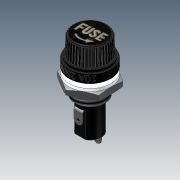
# Autodesk Inventor part: Fuse holder
Saved by Autodesk Inventor 2012 SP2 (Build 160219200, 219)
## iProperties
Created: 2017-11-11
Part Number: Fuse holder
Material: Default
Document SubType Name: Modeling
Designer: Шумейко Д.А.
Density: 1 g/cm^3
Author: Шумейко Д.А.
Autodesk Inventor part; units mm, degrees
sketch "Эскиз1" plane through (0, 0, 0) normal (0, 0, 1) x (1, 0, 0)
  circle A0 centre (0, 0) radius 5.75
  dimension "d0" = 11.5
  constraints: 1 centre point, 1 coincident
  measures "d0" diameter of A0
extrude "Выдавливание1" add sketch "Эскиз1" along normal blind 0.5
ref_plane "РабПлоскость1" through (0, 0, -6) normal (0, 0, -1) x (-1, 0, 0)
sketch "Эскиз2" plane through (0, 0, -6) normal (0, 0, -1) x (-1, 0, 0)
  circle A0 centre (0, 0) radius 6
  dimension "d4" = 12
  constraints: 1 centre point, 1 coincident
  measures "d4" diameter of A0
loft "По сечениям1" add profiles "Эскиз2" section 1 edges at (-5.75, 0, 0)
sketch "Эскиз4" plane through (0, 0, -6) normal (0, 0, -1) x (-1, 0, 0)
  circle A0 centre (0, 0) radius 7
  dimension "d9" = 14
  constraints: 1 centre point, 1 coincident
  measures "d9" diameter of A0
extrude "Выдавливание2" add sketch "Эскиз4" along normal blind 1
sketch "Эскиз5" plane through (0, 0, 0) normal (0, 0, 1) x (1, 0, 0)
  line L0 (-0.3727, 5.7711) -> (-0.0631, 6.1689)
  line L1 (0.0631, 6.1689) -> (0.3727, 5.7711)
  circle A0 centre (0, 0) radius 5.75 projected
  arc A1 (0.0631, 6.1689) -> (-0.0631, 6.1689) centre (0, 6.1198) ccw
  arc A2 (-0.4439, 5.7328) -> (0.4439, 5.7328) centre (0, 0) ccw
  arc A3 (-0.4439, 5.7328) -> (-0.3727, 5.7711) centre (-0.4516, 5.8325) ccw
  arc A4 (0.3727, 5.7711) -> (0.4439, 5.7328) centre (0.4516, 5.8325) ccw
  arc A5 (0.4439, 5.7328) -> (-0.4439, 5.7328) centre (0, 0) ccw
  point P0 (-0.4, 5.7361)
  point P1 (0, 6.25)
  point P2 (0.4, 5.7361)
  point P3 (0, 5.75)
  dimension "d12" = 0.5
  dimension "d13" = 0.8
  dimension "d14" = 0.08
  dimension "d15" = 0.1
  constraints: 16 point on circle, 6 tangent, 5 centre point, 4 end point, 4 point on line, 2 vertical alignment, 1 coincident, 1 equal length, 1 equal radius
  measures "d12" distance of point (0, 6.25) A0.start
  measures "d13" distance of point (0.4, 5.736) A0.end
  measures "d14" radius of A1
  measures "d15" radius of A3
sketch "Эскиз6" plane through (0, 0, 0) normal (1, 0, 0) x (0, 1, 0)
  line L0 (6, -6) -> (5.75, 0) projected
  point P0 (0, 0)
sweep "Сдвиг1" add profiles "Эскиз5" path "Эскиз6" contours L0 A1 L1 A4 A0 A3
sketch "Эскиз7" plane through (0, 0, -7) normal (0, 0, -1) x (-1, 0, 0)
  circle A0 centre (0, 0) radius 7 projected
  circle A1 centre (0, 0) radius 7.5
  dimension "d20" = 15
  constraints: 1 centre point, 1 coincident
  measures "d20" diameter of A1
extrude "Выдавливание3" add sketch "Эскиз7" along normal blind 3 contours A0 | A1
sketch "Эскиз8" plane through (0, 0, 0.5) normal (0, 0, 1) x (1, 0, 0)
  line L0 (-6.3909, 6.5709) -> (6.3606, 6.5709) construction
  line L1 (6.3606, 6.5709) -> (6.3606, -7.9897) construction
  line L2 (6.3606, -7.9897) -> (-6.3909, -7.9897) construction
  line L3 (-6.3909, -7.9897) -> (-6.3909, 6.5709) construction
  constraints: 1 vertical, 2 other
decal "Маркировка1"
fillet "Сопряжение1" radius 0.2 1 edges at (-5.75, 0, 0.5)
pattern_circular "Круговой массив2" count 40 over 360 about axis through (0, 0, -6) along (0, 0, 1) of "Сдвиг1"
sketch "Эскиз9" plane through (0, 0, -10) normal (0, 0, -1) x (-1, 0, 0)
  circle A0 centre (0, 0) radius 7.5 projected
  circle A1 centre (0, 0) radius 5.5
  dimension "d62" = 11
  constraints: 1 centre point, 1 coincident
  measures "d62" diameter of A1
extrude "Выдавливание4" add sketch "Эскиз9" along normal blind 9 contours A1
sketch "Эскиз10" plane through (0, 0, -19) normal (0, 0, -1) x (-1, 0, 0)
  circle A0 centre (0, 0) radius 5.5 projected
  circle A1 centre (0, 0) radius 4
  dimension "d65" = 8
  constraints: 1 centre point, 1 coincident
  measures "d65" diameter of A1
extrude "Выдавливание5" add sketch "Эскиз10" along normal blind 11 contours A1
chamfer "Фаска1" distance 0.5 angle 45 1 edges at (5.5, 0, -19)
thread "Резьба1" size "M11x1.5" class "6g" standard "ANSI Metric M Profile" full length
sketch "Эскиз11" plane through (0, 0, -30) normal (0, 0, -1) x (-1, 0, 0)
  circle A0 centre (0, 0) radius 4 projected
  line L0 (-1.9365, -3.5) -> (1.9365, -3.5)
  dimension "d73" = 3.5
  constraints: 2 end point, 2 point on circle, 1 horizontal
  measures "d73" distance from line of L0 A0.centre
extrude "Выдавливание6" cut sketch "Эскиз11" against normal blind 9 contours L0 A0 picked at (0.3981, -3.6058)
sketch "Эскиз12" plane through (0, 0, -30) normal (0, 0, -1) x (-1, 0, 0)
  arc A0 (1.9365, -3.5) -> (-1.9365, -3.5) centre (0, 0) ccw projected
  line L0 (-1.5, 2.7) -> (1.5, 2.7)
  line L1 (1.5, 2.7) -> (1.5, 2.5)
  line L2 (1.5, 2.5) -> (-1.5, 2.5)
  line L3 (-1.5, 2.5) -> (-1.5, 2.7)
  point P0 (0, 2.5)
  dimension "d76" = 0.2
  dimension "d77" = 3
  dimension "d78" = 2.5
  constraints: 8 end point, 2 parallel, 1 horizontal, 1 midpoint, 1 perpendicular, 1 vertical alignment
  measures "d76" distance of L0.end L1.end
  measures "d77" distance of L0.start L0.end
  measures "d78" distance from line of A0.centre L2
extrude "Выдавливание7" add sketch "Эскиз12" along normal blind 5
fillet "Сопряжение2" radius 1.5 2 edges at (1.5, 2.6, -35) (-1.5, 2.6, -35)
hole "Отверстие1" at (0, 2.5, -33.5) direction (0, 1, 0) diameter 1 end through all
sketch "Эскиз13" plane through (-1.9365, -3.5, -30) normal (0, -1, 0) x (1, 0, 0)
  line L0 (0, 9) -> (3.873, 9) projected
  line L1 (0.4365, 8.9) -> (3.4365, 8.9)
  line L2 (3.4365, 8.9) -> (3.4365, 8.7)
  line L3 (3.4365, 8.7) -> (0.4365, 8.7)
  line L4 (0.4365, 8.7) -> (0.4365, 8.9)
  line L5 (3.873, 9) -> (0, 9) projected
  point P0 (1.9365, 30)
  point P1 (1.9365, 8.9)
  point P2 (1.9365, 9)
  dimension "d91" = 0.2
  dimension "d92" = 3
  dimension "d93" = 0.1
  constraints: 8 end point, 2 midpoint, 2 parallel, 1 horizontal, 1 perpendicular, 1 vertical alignment
  measures "d91" distance of L1.end L2.end
  measures "d92" distance of L2.end L3.end
  measures "d93" distance between parallel lines of L0 L1
sketch "Эскиз14" plane through (0, 0, 0) normal (1, 0, 0) x (0, 1, 0)
  arc A0 (-3.5, -21.1) -> (-4.3, -21.9) centre (-3.5, -21.9) ccw
  line L0 (-4.3, -21.9) -> (-4.3, -25.9)
  point P0 (0, 0)
  dimension "d94" = 0.8
  dimension "d95" = 4
  constraints: 2 end point, 2 point on circle, 1 centre point, 1 horizontal alignment, 1 tangent, 1 vertical, 1 vertical alignment
  measures "d94" radius of A0
  measures "d95" distance of L0.start L0.end
sweep "Сдвиг2" add profiles "Эскиз13" path "Эскиз14"
fillet "Сопряжение3" radius 1.5 2 edges at (1.5, -4.2, -25.9) (-1.5, -4.2, -25.9)
hole "Отверстие2" at (0, -4.3, -24.4) direction (0, 1, 0) diameter 1 depth 0.2 tip angle 118
ref_plane "РабПлоскость2" through (0, 0, -11.5) normal (0, 0, -1) x (-1, 0, 0)
sketch "Эскиз15" plane through (0, 0, -11.5) normal (0, 0, -1) x (-1, 0, 0)
  circle A0 centre (0, 0) radius 7.5 projected
  circle A1 centre (0, 0) radius 5.5 projected
extrude "Выдавливание8" add sketch "Эскиз15" along normal blind 1
sketch "Эскиз16" plane through (0, 0, -12.5) normal (0, 0, -1) x (-1, 0, 0)
  circle A0 centre (0, 0) radius 5.5 projected
  circle A1 centre (0, 0) radius 7.5 projected
  line L0 (0, 8.6603) -> (7.5, 4.3301)
  line L1 (7.5, 4.3301) -> (7.5, -4.3301)
  line L2 (7.5, -4.3301) -> (0, -8.6603)
  line L3 (0, -8.6603) -> (-7.5, -4.3301)
  line L4 (-7.5, -4.3301) -> (-7.5, 4.3301)
  line L5 (-7.5, 4.3301) -> (0, 8.6603)
  dimension "d110" = 15
  constraints: 12 end point, 1 coincident, 1 vertical alignment, 13 other
  measures "d110" distance between parallel lines of L1 L4
extrude "Выдавливание9" add sketch "Эскиз16" along normal blind 2.5
sketch "Эскиз17" plane through (0, 0, 0) normal (1, 0, 0) x (0, 1, 0)
  line L0 (0, 0) -> (0, -44.8004)
  line L1 (8.6603, -12.5) -> (5.6603, -12.5)
  line L2 (8.6603, -15) -> (4.3301, -15) projected
  line L3 (8.6603, -12.5) -> (8.6603, -13)
  line L4 (8.6603, -13) -> (7.1603, -12.5)
  line L5 (8.6603, -12.5) -> (7.1603, -12.5)
  line L6 (8.6603, -15) -> (8.6603, -14.5)
  line L7 (8.6603, -14.5) -> (7.1603, -15)
  line L8 (8.6603, -15) -> (7.1603, -15)
  dimension "d113" = 44.8004
  dimension "d114" = 0.5
  dimension "d115" = 1.5
  dimension "d117" = 0.5
  dimension "d118" = 1.5
  constraints: 16 end point, 3 perpendicular, 1 coincident, 1 collinear, 1 horizontal, 1 midpoint, 1 point on line, 1 vertical
  measures "d113" distance of L0.end L0.start
  measures "d114" distance of L1.start L3.end
  measures "d115" distance from line of L4.end L3
  measures "d117" distance of L2.start L6.end
  measures "d118" distance from line of L7.end L6
revolve "Вращение1" cut sketch "Эскиз17" angle 360 about axis through (0, 0, 0) along (0, 0, -1)
ref_plane "РабПлоскость3" through (0, 9.25, 0) normal (0, 1, 0) x (-1, 0, 0)
sketch "Эскиз18" plane through (0, 9.25, 0) normal (0, 1, 0) x (-1, 0, 0)
  line L0 (7.588, -9.5) -> (-7.412, -9.5) construction
  line L1 (-7.412, -9.5) -> (-7.412, -7.5) construction
  line L2 (-7.412, -7.5) -> (7.588, -7.5) construction
  line L3 (7.588, -7.5) -> (7.588, -9.5) construction
  line L4 (7.5, -10) -> (-7.5, -10) projected
  line L5 (6.3092, -7.4579) -> (7.2849, -7.4579)
  line L6 (7.2849, -7.4579) -> (7.2849, -7.6621)
  line L7 (7.2849, -7.6621) -> (6.9219, -7.6621)
  line L8 (6.9219, -7.6621) -> (6.9219, -9.0024)
  line L9 (6.9219, -9.0024) -> (7.2849, -9.0024)
  line L10 (7.2849, -9.0024) -> (7.2849, -9.1856)
  spline S0 degree 2 poles (7.2849, -9.1856) (7.0791, -9.1856) (6.8846, -9.3023) (6.8716, -9.4643) knots 0 0 0 1 2 2 2
  line L11 (6.8716, -9.4643) -> (6.6642, -9.4643)
  line L12 (6.6642, -9.4643) -> (6.6642, -7.6621)
  line L13 (6.6642, -7.6621) -> (6.3092, -7.6621)
  line L14 (6.3092, -7.6621) -> (6.3092, -7.4579)
  spline S1 degree 2 poles (4.729, -8.0932) (4.729, -7.9489) (4.8214, -7.7026) (4.9057, -7.6118) knots 0 0 0 1 2 2 2
  spline S2 degree 2 poles (4.9057, -7.6118) (4.99, -7.5211) (5.2412, -7.4157) (5.3968, -7.4157) knots 0 0 0 1 2 2 2
  spline S3 degree 2 poles (5.3968, -7.4157) (5.5394, -7.4157) (5.8182, -7.4789) (5.9203, -7.5292) knots 0 0 0 1 2 2 2
  line L15 (5.9203, -7.5292) -> (5.9203, -7.8128)
  line L16 (5.9203, -7.8128) -> (5.9008, -7.8128)
  spline S4 degree 2 poles (5.9008, -7.8128) (5.87, -7.7901) (5.7549, -7.7318) (5.6853, -7.7058) knots 0 0 0 1 2 2 2
  spline S5 degree 2 poles (5.6853, -7.7058) (5.6058, -7.6783) (5.4746, -7.6475) (5.3919, -7.6475) knots 0 0 0 1 2 2 2
  spline S6 degree 2 poles (5.3919, -7.6475) (5.3109, -7.6475) (5.1585, -7.7058) (5.1034, -7.769) knots 0 0 0 1 2 2 2
  spline S7 degree 2 poles (5.1034, -7.769) (5.0532, -7.829) (5.0013, -7.9878) (5.0013, -8.0948) knots 0 0 0 1 2 2 2
  spline S8 degree 2 poles (5.0013, -8.0948) (5.0013, -8.2018) (5.0596, -8.3379) (5.1148, -8.3833) knots 0 0 0 1 2 2 2
  spline S9 degree 2 poles (5.1148, -8.3833) (5.1715, -8.4335) (5.34, -8.4757) (5.4421, -8.4757) knots 0 0 0 1 2 2 2
  spline S10 degree 2 poles (5.4421, -8.4757) (5.5524, -8.4757) (5.7712, -8.4417) (5.8376, -8.4271) knots 0 0 0 1 2 2 2
  line L17 (5.8376, -8.4271) -> (5.8376, -9.4579)
  line L18 (5.8376, -9.4579) -> (4.7404, -9.4579)
  line L19 (4.7404, -9.4579) -> (4.7404, -9.2229)
  line L20 (4.7404, -9.2229) -> (5.5799, -9.2229)
  line L21 (5.5799, -9.2229) -> (5.5799, -8.6896)
  spline S11 degree 2 poles (5.5799, -8.6896) (5.5313, -8.6961) (5.4373, -8.701) (5.3984, -8.701) knots 0 0 0 1 2 2 2
  spline S12 degree 2 poles (5.3984, -8.701) (5.2444, -8.701) (5.0321, -8.6507) (4.9349, -8.5762) knots 0 0 0 1 2 2 2
  spline S13 degree 2 poles (4.9349, -8.5762) (4.836, -8.5016) (4.729, -8.2747) (4.729, -8.0932) knots 0 0 0 1 2 2 2
  line L22 (4.5994, -7.4579) -> (3.9251, -9.4579)
  line L23 (3.9251, -9.4579) -> (3.5977, -9.4579)
  line L24 (3.5977, -9.4579) -> (2.9235, -7.4579)
  line L25 (2.9235, -7.4579) -> (3.2039, -7.4579)
  line L26 (3.2039, -7.4579) -> (3.3854, -8.017)
  line L27 (3.3854, -8.017) -> (4.1488, -8.017)
  line L28 (4.1488, -8.017) -> (4.3303, -7.4579)
  line L29 (4.3303, -7.4579) -> (4.5994, -7.4579)
  line L30 (3.4584, -8.2439) -> (3.7679, -9.1856)
  line L31 (3.7679, -9.1856) -> (4.0759, -8.2439)
  line L32 (4.0759, -8.2439) -> (3.4584, -8.2439)
  line L33 (0.7987, -7.4579) -> (1.7744, -7.4579)
  line L34 (1.7744, -7.4579) -> (1.7744, -7.6621)
  line L35 (1.7744, -7.6621) -> (1.4114, -7.6621)
  line L36 (1.4114, -7.6621) -> (1.4114, -9.0024)
  line L37 (1.4114, -9.0024) -> (1.7744, -9.0024)
  line L38 (1.7744, -9.0024) -> (1.7744, -9.1856)
  spline S14 degree 2 poles (1.7744, -9.1856) (1.5686, -9.1856) (1.3741, -9.3023) (1.3611, -9.4643) knots 0 0 0 1 2 2 2
  line L39 (1.3611, -9.4643) -> (1.1537, -9.4643)
  line L40 (1.1537, -9.4643) -> (1.1537, -7.6621)
  line L41 (1.1537, -7.6621) -> (0.7987, -7.6621)
  line L42 (0.7987, -7.6621) -> (0.7987, -7.4579)
  line L43 (-0.8026, -7.4579) -> (0.4308, -7.4579)
  line L44 (0.4308, -7.4579) -> (0.4308, -7.7415)
  spline S15 degree 2 poles (0.4308, -7.7415) (0.2979, -7.8663) (0.0613, -8.0981) (-0.0522, -8.2229) knots 0 0 0 1 2 2 2
  spline S16 degree 2 poles (-0.0522, -8.2229) (-0.2807, -8.4741) (-0.4476, -8.7755) (-0.4476, -8.936) knots 0 0 0 1 2 2 2
  spline S17 degree 2 poles (-0.4476, -8.936) (-0.4476, -9.0203) (-0.3958, -9.1467) (-0.3488, -9.1872) knots 0 0 0 1 2 2 2
  spline S18 degree 2 poles (-0.3488, -9.1872) (-0.3018, -9.2277) (-0.1786, -9.2682) (-0.104, -9.2682) knots 0 0 0 1 2 2 2
  spline S19 degree 2 poles (-0.104, -9.2682) (-0.0327, -9.2682) (0.1131, -9.2326) (0.1796, -9.205) knots 0 0 0 1 2 2 2
  spline S20 degree 2 poles (0.1796, -9.205) (0.2363, -9.1823) (0.3417, -9.1175) (0.3741, -9.0948) knots 0 0 0 1 2 2 2
  line L45 (0.3741, -9.0948) -> (0.3887, -9.0948)
  line L46 (0.3887, -9.0948) -> (0.3887, -9.3801)
  spline S21 degree 2 poles (0.3887, -9.3801) (0.306, -9.4206) (0.0094, -9.5) (-0.1235, -9.5) knots 0 0 0 1 2 2 2
  spline S22 degree 2 poles (-0.1235, -9.5) (-0.4039, -9.5) (-0.7199, -9.2034) (-0.7199, -8.9506) knots 0 0 0 1 2 2 2
  spline S23 degree 2 poles (-0.7199, -8.9506) (-0.7199, -8.8323) (-0.6648, -8.6345) (-0.6162, -8.5502) knots 0 0 0 1 2 2 2
  spline S24 degree 2 poles (-0.6162, -8.5502) (-0.5676, -8.4627) (-0.4266, -8.2909) (-0.3488, -8.2083) knots 0 0 0 1 2 2 2
  spline S25 degree 2 poles (-0.3488, -8.2083) (-0.2224, -8.0705) (0.0872, -7.7755) (0.1796, -7.6896) knots 0 0 0 1 2 2 2
  line L47 (0.1796, -7.6896) -> (-0.8026, -7.6896)
  line L48 (-0.8026, -7.6896) -> (-0.8026, -7.4579)
  spline S26 degree 2 poles (-2.2823, -8.0932) (-2.2823, -7.9489) (-2.1899, -7.7026) (-2.1057, -7.6118) knots 0 0 0 1 2 2 2
  spline S27 degree 2 poles (-2.1057, -7.6118) (-2.0214, -7.5211) (-1.7702, -7.4157) (-1.6146, -7.4157) knots 0 0 0 1 2 2 2
  spline S28 degree 2 poles (-1.6146, -7.4157) (-1.472, -7.4157) (-1.1932, -7.4789) (-1.0911, -7.5292) knots 0 0 0 1 2 2 2
  line L49 (-1.0911, -7.5292) -> (-1.0911, -7.8128)
  line L50 (-1.0911, -7.8128) -> (-1.1105, -7.8128)
  spline S29 degree 2 poles (-1.1105, -7.8128) (-1.1413, -7.7901) (-1.2564, -7.7318) (-1.3261, -7.7058) knots 0 0 0 1 2 2 2
  spline S30 degree 2 poles (-1.3261, -7.7058) (-1.4055, -7.6783) (-1.5368, -7.6475) (-1.6194, -7.6475) knots 0 0 0 1 2 2 2
  spline S31 degree 2 poles (-1.6194, -7.6475) (-1.7005, -7.6475) (-1.8528, -7.7058) (-1.9079, -7.769) knots 0 0 0 1 2 2 2
  spline S32 degree 2 poles (-1.9079, -7.769) (-1.9582, -7.829) (-2.01, -7.9878) (-2.01, -8.0948) knots 0 0 0 1 2 2 2
  spline S33 degree 2 poles (-2.01, -8.0948) (-2.01, -8.2018) (-1.9517, -8.3379) (-1.8966, -8.3833) knots 0 0 0 1 2 2 2
  spline S34 degree 2 poles (-1.8966, -8.3833) (-1.8399, -8.4335) (-1.6713, -8.4757) (-1.5692, -8.4757) knots 0 0 0 1 2 2 2
  spline S35 degree 2 poles (-1.5692, -8.4757) (-1.459, -8.4757) (-1.2402, -8.4417) (-1.1737, -8.4271) knots 0 0 0 1 2 2 2
  line L51 (-1.1737, -8.4271) -> (-1.1737, -9.4579)
  line L52 (-1.1737, -9.4579) -> (-2.271, -9.4579)
  line L53 (-2.271, -9.4579) -> (-2.271, -9.2229)
  line L54 (-2.271, -9.2229) -> (-1.4314, -9.2229)
  line L55 (-1.4314, -9.2229) -> (-1.4314, -8.6896)
  spline S36 degree 2 poles (-1.4314, -8.6896) (-1.4801, -8.6961) (-1.5741, -8.701) (-1.613, -8.701) knots 0 0 0 1 2 2 2
  spline S37 degree 2 poles (-1.613, -8.701) (-1.7669, -8.701) (-1.9792, -8.6507) (-2.0765, -8.5762) knots 0 0 0 1 2 2 2
  spline S38 degree 2 poles (-2.0765, -8.5762) (-2.1754, -8.5016) (-2.2823, -8.2747) (-2.2823, -8.0932) knots 0 0 0 1 2 2 2
  line L56 (-4.0781, -9.4579) -> (-3.3893, -7.4579)
  line L57 (-3.3893, -7.4579) -> (-3.1024, -7.4579)
  line L58 (-3.1024, -7.4579) -> (-2.4136, -9.4579)
  line L59 (-2.4136, -9.4579) -> (-2.6989, -9.4579)
  line L60 (-2.6989, -9.4579) -> (-3.2532, -7.7966)
  line L61 (-3.2532, -7.7966) -> (-3.8075, -9.4579)
  line L62 (-3.8075, -9.4579) -> (-4.0781, -9.4579)
  line L63 (-4.0538, -7.4579) -> (-4.728, -9.4579)
  line L64 (-4.728, -9.4579) -> (-5.0554, -9.4579)
  line L65 (-5.0554, -9.4579) -> (-5.7297, -7.4579)
  line L66 (-5.7297, -7.4579) -> (-5.4493, -7.4579)
  line L67 (-5.4493, -7.4579) -> (-5.2677, -8.017)
  line L68 (-5.2677, -8.017) -> (-4.5044, -8.017)
  line L69 (-4.5044, -8.017) -> (-4.3228, -7.4579)
  line L70 (-4.3228, -7.4579) -> (-4.0538, -7.4579)
  line L71 (-5.1948, -8.2439) -> (-4.8852, -9.1856)
  line L72 (-4.8852, -9.1856) -> (-4.5773, -8.2439)
  line L73 (-4.5773, -8.2439) -> (-5.1948, -8.2439)
  spline S39 degree 2 poles (-6.7005, -7.4222) (-6.506, -7.4222) (-6.177, -7.5535) (-6.057, -7.6848) knots 0 0 0 1 2 2 2
  spline S40 degree 2 poles (-6.057, -7.6848) (-5.9371, -7.8144) (-5.8058, -8.2034) (-5.8058, -8.4562) knots 0 0 0 1 2 2 2
  spline S41 degree 2 poles (-5.8058, -8.4562) (-5.8058, -8.7075) (-5.9339, -9.0802) (-6.0554, -9.218) knots 0 0 0 1 2 2 2
  spline S42 degree 2 poles (-6.0554, -9.218) (-6.1754, -9.3525) (-6.5028, -9.4935) (-6.7053, -9.4935) knots 0 0 0 1 2 2 2
  spline S43 degree 2 poles (-6.7053, -9.4935) (-6.8058, -9.4935) (-6.9825, -9.4643) (-7.057, -9.4417) knots 0 0 0 1 2 2 2
  spline S44 degree 2 poles (-7.057, -9.4417) (-7.1219, -9.4206) (-7.2564, -9.3606) (-7.3228, -9.325) knots 0 0 0 1 2 2 2
  line L74 (-7.3228, -9.325) -> (-7.3228, -9.0041)
  line L75 (-7.3228, -9.0041) -> (-7.3018, -9.0041)
  spline S45 degree 2 poles (-7.3018, -9.0041) (-7.2661, -9.0365) (-7.1559, -9.1272) (-7.0765, -9.171) knots 0 0 0 1 2 2 2
  spline S46 degree 2 poles (-7.0765, -9.171) (-7.0003, -9.2131) (-6.8204, -9.2666) (-6.7037, -9.2666) knots 0 0 0 1 2 2 2
  spline S47 degree 2 poles (-6.7037, -9.2666) (-6.5757, -9.2666) (-6.3472, -9.1613) (-6.2613, -9.0608) knots 0 0 0 1 2 2 2
  spline S48 degree 2 poles (-6.2613, -9.0608) (-6.177, -8.9587) (-6.083, -8.6491) (-6.083, -8.4562) knots 0 0 0 1 2 2 2
  spline S49 degree 2 poles (-6.083, -8.4562) (-6.083, -8.2504) (-6.1818, -7.9538) (-6.2677, -7.8517) knots 0 0 0 1 2 2 2
  spline S50 degree 2 poles (-6.2677, -7.8517) (-6.352, -7.7528) (-6.5773, -7.6523) (-6.7037, -7.6523) knots 0 0 0 1 2 2 2
  spline S51 degree 2 poles (-6.7037, -7.6523) (-6.8188, -7.6523) (-7.0149, -7.7091) (-7.0911, -7.7512) knots 0 0 0 1 2 2 2
  spline S52 degree 2 poles (-7.0911, -7.7512) (-7.164, -7.7934) (-7.2726, -7.8809) (-7.3034, -7.9117) knots 0 0 0 1 2 2 2
  line L76 (-7.3034, -7.9117) -> (-7.3228, -7.9117)
  line L77 (-7.3228, -7.9117) -> (-7.3228, -7.594)
  spline S53 degree 2 poles (-7.3228, -7.594) (-7.2564, -7.5632) (-7.1397, -7.5065) (-7.057, -7.4806) knots 0 0 0 1 2 2 2
  spline S54 degree 2 poles (-7.057, -7.4806) (-6.9695, -7.4514) (-6.8204, -7.4222) (-6.7005, -7.4222) knots 0 0 0 1 2 2 2
  point P0 (0, 0)
  dimension "d121" = 15
  dimension "d122" = 2
  dimension "d124" = 0.5
  constraints: 1 horizontal, 2 other
  measures "d121" distance of L1.end L2.end
  measures "d122" distance of L2.end L0.start
  measures "d124" distance between parallel lines of L4 L0
emboss "Рельеф1" sketch "Эскиз18" operation add depth 0.1 direction (0, 1, 0) wrap yes faces at (-7.4757, -0.6035, -9)
ref_plane "РабПлоскость4" through (0, -10, 0) normal (0, -1, 0) x (1, 0, 0)
sketch "Эскиз19" plane through (0, -10, 0) normal (0, -1, 0) x (1, 0, 0)
  line L0 (7.6141, -9.5) -> (-7.3422, -9.5) construction
  line L1 (-7.3422, -9.5) -> (-7.3422, -7.4157) construction
  line L2 (-7.3422, -7.4157) -> (7.6141, -7.4157) construction
  line L3 (7.6141, -7.4157) -> (7.6141, -9.5) construction
  line L4 (7.5, -10) -> (-7.5, -10) projected
  line L5 (6.3353, -7.4579) -> (7.311, -7.4579)
  line L6 (7.311, -7.4579) -> (7.311, -7.6621)
  line L7 (7.311, -7.6621) -> (6.948, -7.6621)
  line L8 (6.948, -7.6621) -> (6.948, -9.0024)
  line L9 (6.948, -9.0024) -> (7.311, -9.0024)
  line L10 (7.311, -9.0024) -> (7.311, -9.1856)
  spline S0 degree 2 poles (7.311, -9.1856) (7.1052, -9.1856) (6.9107, -9.3023) (6.8977, -9.4643) knots 0 0 0 1 2 2 2
  line L11 (6.8977, -9.4643) -> (6.6903, -9.4643)
  line L12 (6.6903, -9.4643) -> (6.6903, -7.6621)
  line L13 (6.6903, -7.6621) -> (6.3353, -7.6621)
  line L14 (6.3353, -7.6621) -> (6.3353, -7.4579)
  spline S1 degree 2 poles (4.7227, -8.4579) (4.7227, -7.9198) (5.0355, -7.4157) (5.3612, -7.4157) knots 0 0 0 1 2 2 2
  spline S2 degree 2 poles (5.3612, -7.4157) (5.6919, -7.4157) (6.0014, -7.9295) (6.0014, -8.4562) knots 0 0 0 1 2 2 2
  spline S3 degree 2 poles (6.0014, -8.4562) (6.0014, -8.9976) (5.6886, -9.4984) (5.3612, -9.4984) knots 0 0 0 1 2 2 2
  spline S4 degree 2 poles (5.3612, -9.4984) (5.0322, -9.4984) (4.7227, -8.9797) (4.7227, -8.4579) knots 0 0 0 1 2 2 2
  spline S5 degree 2 poles (5.0663, -7.8485) (5.0274, -7.9473) (4.995, -8.252) (4.995, -8.4579) knots 0 0 0 1 2 2 2
  spline S6 degree 2 poles (4.995, -8.4579) (4.995, -8.6637) (5.0274, -8.9668) (5.0679, -9.0689) knots 0 0 0 1 2 2 2
  spline S7 degree 2 poles (5.0679, -9.0689) (5.1084, -9.171) (5.2494, -9.2763) (5.3612, -9.2763) knots 0 0 0 1 2 2 2
  spline S8 degree 2 poles (5.3612, -9.2763) (5.4731, -9.2763) (5.6173, -9.171) (5.6595, -9.0656) knots 0 0 0 1 2 2 2
  spline S9 degree 2 poles (5.6595, -9.0656) (5.7, -8.9635) (5.7292, -8.6524) (5.7292, -8.4562) knots 0 0 0 1 2 2 2
  spline S10 degree 2 poles (5.7292, -8.4562) (5.7292, -8.2455) (5.7032, -7.9635) (5.6611, -7.8533) knots 0 0 0 1 2 2 2
  spline S11 degree 2 poles (5.6611, -7.8533) (5.6222, -7.7496) (5.4779, -7.6378) (5.3612, -7.6378) knots 0 0 0 1 2 2 2
  spline S12 degree 2 poles (5.3612, -7.6378) (5.251, -7.6378) (5.1068, -7.7431) (5.0663, -7.8485) knots 0 0 0 1 2 2 2
  line L15 (4.6254, -7.4579) -> (3.9512, -9.4579)
  line L16 (3.9512, -9.4579) -> (3.6238, -9.4579)
  line L17 (3.6238, -9.4579) -> (2.9496, -7.4579)
  line L18 (2.9496, -7.4579) -> (3.23, -7.4579)
  line L19 (3.23, -7.4579) -> (3.4115, -8.017)
  line L20 (3.4115, -8.017) -> (4.1749, -8.017)
  line L21 (4.1749, -8.017) -> (4.3564, -7.4579)
  line L22 (4.3564, -7.4579) -> (4.6254, -7.4579)
  line L23 (3.4844, -8.2439) -> (3.794, -9.1856)
  line L24 (3.794, -9.1856) -> (4.1019, -8.2439)
  line L25 (4.1019, -8.2439) -> (3.4844, -8.2439)
  line L26 (0.7243, -7.4579) -> (1.9577, -7.4579)
  line L27 (1.9577, -7.4579) -> (1.9577, -7.7415)
  spline S13 degree 2 poles (1.9577, -7.7415) (1.8248, -7.8663) (1.5882, -8.0981) (1.4747, -8.2229) knots 0 0 0 1 2 2 2
  spline S14 degree 2 poles (1.4747, -8.2229) (1.2462, -8.4741) (1.0792, -8.7755) (1.0792, -8.936) knots 0 0 0 1 2 2 2
  spline S15 degree 2 poles (1.0792, -8.936) (1.0792, -9.0203) (1.1311, -9.1467) (1.1781, -9.1872) knots 0 0 0 1 2 2 2
  spline S16 degree 2 poles (1.1781, -9.1872) (1.2251, -9.2277) (1.3483, -9.2682) (1.4228, -9.2682) knots 0 0 0 1 2 2 2
  spline S17 degree 2 poles (1.4228, -9.2682) (1.4942, -9.2682) (1.64, -9.2326) (1.7065, -9.205) knots 0 0 0 1 2 2 2
  spline S18 degree 2 poles (1.7065, -9.205) (1.7632, -9.1823) (1.8685, -9.1175) (1.901, -9.0948) knots 0 0 0 1 2 2 2
  line L28 (1.901, -9.0948) -> (1.9155, -9.0948)
  line L29 (1.9155, -9.0948) -> (1.9155, -9.3801)
  spline S19 degree 2 poles (1.9155, -9.3801) (1.8329, -9.4206) (1.5363, -9.5) (1.4034, -9.5) knots 0 0 0 1 2 2 2
  spline S20 degree 2 poles (1.4034, -9.5) (1.123, -9.5) (0.807, -9.2034) (0.807, -8.9506) knots 0 0 0 1 2 2 2
  spline S21 degree 2 poles (0.807, -8.9506) (0.807, -8.8323) (0.8621, -8.6345) (0.9107, -8.5502) knots 0 0 0 1 2 2 2
  spline S22 degree 2 poles (0.9107, -8.5502) (0.9593, -8.4627) (1.1003, -8.2909) (1.1781, -8.2083) knots 0 0 0 1 2 2 2
  spline S23 degree 2 poles (1.1781, -8.2083) (1.3045, -8.0705) (1.6141, -7.7755) (1.7065, -7.6896) knots 0 0 0 1 2 2 2
  line L30 (1.7065, -7.6896) -> (0.7243, -7.6896)
  line L31 (0.7243, -7.6896) -> (0.7243, -7.4579)
  spline S24 degree 2 poles (-0.7554, -8.0932) (-0.7554, -7.9489) (-0.6631, -7.7026) (-0.5788, -7.6118) knots 0 0 0 1 2 2 2
  spline S25 degree 2 poles (-0.5788, -7.6118) (-0.4945, -7.5211) (-0.2433, -7.4157) (-0.0877, -7.4157) knots 0 0 0 1 2 2 2
  spline S26 degree 2 poles (-0.0877, -7.4157) (0.0549, -7.4157) (0.3337, -7.4789) (0.4358, -7.5292) knots 0 0 0 1 2 2 2
  line L32 (0.4358, -7.5292) -> (0.4358, -7.8128)
  line L33 (0.4358, -7.8128) -> (0.4164, -7.8128)
  spline S27 degree 2 poles (0.4164, -7.8128) (0.3856, -7.7901) (0.2705, -7.7318) (0.2008, -7.7058) knots 0 0 0 1 2 2 2
  spline S28 degree 2 poles (0.2008, -7.7058) (0.1214, -7.6783) (-0.0099, -7.6475) (-0.0926, -7.6475) knots 0 0 0 1 2 2 2
  spline S29 degree 2 poles (-0.0926, -7.6475) (-0.1736, -7.6475) (-0.3259, -7.7058) (-0.3811, -7.769) knots 0 0 0 1 2 2 2
  spline S30 degree 2 poles (-0.3811, -7.769) (-0.4313, -7.829) (-0.4832, -7.9878) (-0.4832, -8.0948) knots 0 0 0 1 2 2 2
  spline S31 degree 2 poles (-0.4832, -8.0948) (-0.4832, -8.2018) (-0.4248, -8.3379) (-0.3697, -8.3833) knots 0 0 0 1 2 2 2
  spline S32 degree 2 poles (-0.3697, -8.3833) (-0.313, -8.4335) (-0.1444, -8.4757) (-0.0423, -8.4757) knots 0 0 0 1 2 2 2
  spline S33 degree 2 poles (-0.0423, -8.4757) (0.0679, -8.4757) (0.2867, -8.4417) (0.3531, -8.4271) knots 0 0 0 1 2 2 2
  line L34 (0.3531, -8.4271) -> (0.3531, -9.4579)
  line L35 (0.3531, -9.4579) -> (-0.7441, -9.4579)
  line L36 (-0.7441, -9.4579) -> (-0.7441, -9.2229)
  line L37 (-0.7441, -9.2229) -> (0.0954, -9.2229)
  line L38 (0.0954, -9.2229) -> (0.0954, -8.6896)
  spline S34 degree 2 poles (0.0954, -8.6896) (0.0468, -8.6961) (-0.0472, -8.701) (-0.0861, -8.701) knots 0 0 0 1 2 2 2
  spline S35 degree 2 poles (-0.0861, -8.701) (-0.24, -8.701) (-0.4524, -8.6507) (-0.5496, -8.5762) knots 0 0 0 1 2 2 2
  spline S36 degree 2 poles (-0.5496, -8.5762) (-0.6485, -8.5016) (-0.7554, -8.2747) (-0.7554, -8.0932) knots 0 0 0 1 2 2 2
  spline S37 degree 2 poles (-2.2887, -8.4579) (-2.2887, -7.9198) (-1.9759, -7.4157) (-1.6501, -7.4157) knots 0 0 0 1 2 2 2
  spline S38 degree 2 poles (-1.6501, -7.4157) (-1.3195, -7.4157) (-1.0099, -7.9295) (-1.0099, -8.4562) knots 0 0 0 1 2 2 2
  spline S39 degree 2 poles (-1.0099, -8.4562) (-1.0099, -8.9976) (-1.3227, -9.4984) (-1.6501, -9.4984) knots 0 0 0 1 2 2 2
  spline S40 degree 2 poles (-1.6501, -9.4984) (-1.9791, -9.4984) (-2.2887, -8.9797) (-2.2887, -8.4579) knots 0 0 0 1 2 2 2
  spline S41 degree 2 poles (-1.9451, -7.8485) (-1.984, -7.9473) (-2.0164, -8.252) (-2.0164, -8.4579) knots 0 0 0 1 2 2 2
  spline S42 degree 2 poles (-2.0164, -8.4579) (-2.0164, -8.6637) (-1.984, -8.9668) (-1.9435, -9.0689) knots 0 0 0 1 2 2 2
  spline S43 degree 2 poles (-1.9435, -9.0689) (-1.9029, -9.171) (-1.7619, -9.2763) (-1.6501, -9.2763) knots 0 0 0 1 2 2 2
  spline S44 degree 2 poles (-1.6501, -9.2763) (-1.5383, -9.2763) (-1.394, -9.171) (-1.3519, -9.0656) knots 0 0 0 1 2 2 2
  spline S45 degree 2 poles (-1.3519, -9.0656) (-1.3114, -8.9635) (-1.2822, -8.6524) (-1.2822, -8.4562) knots 0 0 0 1 2 2 2
  spline S46 degree 2 poles (-1.2822, -8.4562) (-1.2822, -8.2455) (-1.3081, -7.9635) (-1.3503, -7.8533) knots 0 0 0 1 2 2 2
  spline S47 degree 2 poles (-1.3503, -7.8533) (-1.3892, -7.7496) (-1.5334, -7.6378) (-1.6501, -7.6378) knots 0 0 0 1 2 2 2
  spline S48 degree 2 poles (-1.6501, -7.6378) (-1.7603, -7.6378) (-1.9046, -7.7431) (-1.9451, -7.8485) knots 0 0 0 1 2 2 2
  line L39 (-4.052, -9.4579) -> (-3.3632, -7.4579)
  line L40 (-3.3632, -7.4579) -> (-3.0764, -7.4579)
  line L41 (-3.0764, -7.4579) -> (-2.3875, -9.4579)
  line L42 (-2.3875, -9.4579) -> (-2.6728, -9.4579)
  line L43 (-2.6728, -9.4579) -> (-3.2271, -7.7966)
  line L44 (-3.2271, -7.7966) -> (-3.7814, -9.4579)
  line L45 (-3.7814, -9.4579) -> (-4.052, -9.4579)
  line L46 (-4.0277, -7.4579) -> (-4.702, -9.4579)
  line L47 (-4.702, -9.4579) -> (-5.0294, -9.4579)
  line L48 (-5.0294, -9.4579) -> (-5.7036, -7.4579)
  line L49 (-5.7036, -7.4579) -> (-5.4232, -7.4579)
  line L50 (-5.4232, -7.4579) -> (-5.2417, -8.017)
  line L51 (-5.2417, -8.017) -> (-4.4783, -8.017)
  line L52 (-4.4783, -8.017) -> (-4.2968, -7.4579)
  line L53 (-4.2968, -7.4579) -> (-4.0277, -7.4579)
  line L54 (-5.1687, -8.2439) -> (-4.8592, -9.1856)
  line L55 (-4.8592, -9.1856) -> (-4.5512, -8.2439)
  line L56 (-4.5512, -8.2439) -> (-5.1687, -8.2439)
  spline S49 degree 2 poles (-6.6744, -7.4222) (-6.4799, -7.4222) (-6.1509, -7.5535) (-6.031, -7.6848) knots 0 0 0 1 2 2 2
  spline S50 degree 2 poles (-6.031, -7.6848) (-5.911, -7.8144) (-5.7798, -8.2034) (-5.7798, -8.4562) knots 0 0 0 1 2 2 2
  spline S51 degree 2 poles (-5.7798, -8.4562) (-5.7798, -8.7075) (-5.9078, -9.0802) (-6.0294, -9.218) knots 0 0 0 1 2 2 2
  spline S52 degree 2 poles (-6.0294, -9.218) (-6.1493, -9.3525) (-6.4767, -9.4935) (-6.6793, -9.4935) knots 0 0 0 1 2 2 2
  spline S53 degree 2 poles (-6.6793, -9.4935) (-6.7798, -9.4935) (-6.9564, -9.4643) (-7.031, -9.4417) knots 0 0 0 1 2 2 2
  spline S54 degree 2 poles (-7.031, -9.4417) (-7.0958, -9.4206) (-7.2303, -9.3606) (-7.2968, -9.325) knots 0 0 0 1 2 2 2
  line L57 (-7.2968, -9.325) -> (-7.2968, -9.0041)
  line L58 (-7.2968, -9.0041) -> (-7.2757, -9.0041)
  spline S55 degree 2 poles (-7.2757, -9.0041) (-7.24, -9.0365) (-7.1298, -9.1272) (-7.0504, -9.171) knots 0 0 0 1 2 2 2
  spline S56 degree 2 poles (-7.0504, -9.171) (-6.9742, -9.2131) (-6.7943, -9.2666) (-6.6776, -9.2666) knots 0 0 0 1 2 2 2
  spline S57 degree 2 poles (-6.6776, -9.2666) (-6.5496, -9.2666) (-6.3211, -9.1613) (-6.2352, -9.0608) knots 0 0 0 1 2 2 2
  spline S58 degree 2 poles (-6.2352, -9.0608) (-6.1509, -8.9587) (-6.0569, -8.6491) (-6.0569, -8.4562) knots 0 0 0 1 2 2 2
  spline S59 degree 2 poles (-6.0569, -8.4562) (-6.0569, -8.2504) (-6.1558, -7.9538) (-6.2417, -7.8517) knots 0 0 0 1 2 2 2
  spline S60 degree 2 poles (-6.2417, -7.8517) (-6.3259, -7.7528) (-6.5512, -7.6523) (-6.6776, -7.6523) knots 0 0 0 1 2 2 2
  spline S61 degree 2 poles (-6.6776, -7.6523) (-6.7927, -7.6523) (-6.9888, -7.7091) (-7.065, -7.7512) knots 0 0 0 1 2 2 2
  spline S62 degree 2 poles (-7.065, -7.7512) (-7.1379, -7.7934) (-7.2465, -7.8809) (-7.2773, -7.9117) knots 0 0 0 1 2 2 2
  line L59 (-7.2773, -7.9117) -> (-7.2968, -7.9117)
  line L60 (-7.2968, -7.9117) -> (-7.2968, -7.594)
  spline S63 degree 2 poles (-7.2968, -7.594) (-7.2303, -7.5632) (-7.1136, -7.5065) (-7.031, -7.4806) knots 0 0 0 1 2 2 2
  spline S64 degree 2 poles (-7.031, -7.4806) (-6.9435, -7.4514) (-6.7943, -7.4222) (-6.6744, -7.4222) knots 0 0 0 1 2 2 2
  point P0 (0, 0)
  dimension "d128" = 2.0843
  dimension "d129" = 14.9562
  dimension "d130" = 0.5
  constraints: 1 horizontal, 2 other
  measures "d128" distance of L0.end L1.end
  measures "d129" distance of L0.start L0.end
  measures "d130" distance between parallel lines of L0 L4
emboss "Рельеф2" sketch "Эскиз19" operation add depth 0.1 direction (0, -1, 0) wrap yes faces at (-7.0168, 2.6486, -8.6675)
equation "\"d118\" = d115"
